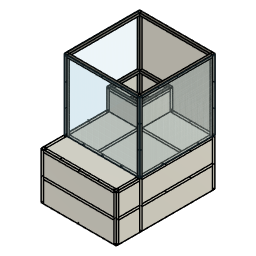
main v17 (Autodesk Fusion 360 design; units mm, degrees)
Autodesk Fusion 360 part; units mm, degrees
note: some values were not read from the file. Chosen so that the rebuilt part matches the saved one: which bodies a step acts on; which face or edge a step refers to.
(part 1 of 2)
sketch "Sketch1" plane through (0, 0, 0) normal (0, 0, 1) x (1, 0, 0) in component "Frame"
  line L0 (0, 0) -> (640, 0)
  line L1 (640, 0) -> (640, 640)
  line L2 (640, 640) -> (0, 640)
  line L3 (0, 640) -> (0, 0)
  line L4 (20, 640) -> (20, 0)
  line L5 (0, 20) -> (640, 20)
  line L6 (620, 640) -> (620, 0)
  line L7 (640, 620) -> (0, 620)
  line L8 (0, 0) -> (0, -200)
  line L9 (0, -200) -> (640, -200)
  line L10 (640, -200) -> (640, 0)
  line L11 (20, 0) -> (20, -200)
  line L12 (620, 0) -> (620, -200)
  line L13 (0, -180) -> (640, -180)
  line L14 (270, 620) -> (270, 20) construction
  line L15 (20, 370) -> (620, 370) construction
  line L16 (280, 620) -> (280, 20)
  line L17 (260, 620) -> (260, 20)
  line L18 (20, 380) -> (620, 380)
  line L19 (20, 360) -> (620, 360)
  line L20 (20, 380) -> (0, 380)
  line L21 (20, 360) -> (0, 360)
  line L22 (260, 620) -> (260, 640)
  line L23 (280, 620) -> (280, 640)
  dimension "d44" = 640
  dimension "d45" = 20
  dimension "d46" = 20
  dimension "d47" = 20
  dimension "d48" = 20
  dimension "d54" = 200
  dimension "d55" = 20
  dimension "d64" = 10
  dimension "d65" = 10
  dimension "d66" = 10
  dimension "d67" = 20
  dimension "d95" = 250
  dimension "d96" = 250
  constraint horizontal L0
  constraint vertical L1
  constraint horizontal L2
  constraint vertical L3
  constraint coincident L0.start L3.end
  constraint equal L0 L3
  constraint coincident L2 L4.start
  constraint coincident L0 L4.end
  constraint perpendicular L0 L4
  constraint coincident L3 L5.start
  constraint coincident L1 L5.end
  constraint perpendicular L1 L5
  constraint coincident L2 L6.start
  constraint coincident L0 L6.end
  constraint perpendicular L0 L6
  constraint coincident L1 L7.start
  constraint coincident L3 L7.end
  constraint perpendicular L3 L7
  constraint vertical L8
  constraint perpendicular L8 L9
  constraint vertical L10
  constraint coincident L9 L11.end
  constraint perpendicular L9 L11
  constraint coincident L9 L12.end
  constraint perpendicular L9 L12
  constraint coincident L8 L13.start
  constraint coincident L10 L13.end
  constraint perpendicular L10 L13
  constraint coincident L7 L16.start
  constraint coincident L5 L16.end
  constraint perpendicular L5 L16
  constraint coincident L7 L17.start
  constraint coincident L5 L17.end
  constraint perpendicular L5 L17
  constraint coincident L4 L18.start
  constraint coincident L6 L18.end
  constraint perpendicular L6 L18
  constraint coincident L4 L19.start
  constraint coincident L6 L19.end
  constraint perpendicular L6 L19
  constraint coincident L4 L15.start
  constraint coincident L6 L15.end
  constraint coincident L5 L14.end
  constraint coincident L7 L14.start
  constraint coincident L3 L20.end
  constraint perpendicular L3 L20
  constraint coincident L3 L21.end
  constraint perpendicular L3 L21
  constraint coincident L2 L22.end
  constraint perpendicular L2 L22
  constraint coincident L2 L23.end
  constraint perpendicular L2 L23
  measures "d44" distance of L0.start L2.end
  measures "d45" distance of L2 L7
  measures "d46" distance of L0 L5
  measures "d47" distance of L3 L4
  measures "d48" distance of L1 L6
  measures "d54" distance of L0.start L8.end
  measures "d55" distance of L9 L13
  measures "d64" distance of L15 L19
  measures "d65" distance of L15 L18
  measures "d66" distance of L14 L16
  measures "d67" distance of L16 L17
  measures "d95" distance of L4 L14
  measures "d96" distance of L7 L15
extrude "Extrude1" add sketch "Sketch1" along normal blind 1000 contours L0 L3 L4 L5 | L0 L1 L5 L6 | L2 L3 L4 L7 | L1 L2 L6 L7 makes body 1 at (0, 633.3333, 333.3333) makes body 2 at (633.3333, 620, 333.3333) makes body 3 at (0, 13.3333, 333.3333) makes body 4 at (620, 13.3333, 333.3333) in component "Frame"
extrude "Extrude6" add sketch "Sketch1" against normal blind 20 from surface at 1000 separate body contours L3 L4 L5 L21 | L3 L4 L20 L21 | L3 L4 L7 L20 makes body 5 in component "Frame"
extrude "Extrude7" add sketch "Sketch1" against normal blind 20 from surface at 1000 separate body contours L2 L4 L7 L22 | L2 L6 L7 L23 | L2 L7 L22 L23 makes body 6 in component "Frame"
extrude "Extrude8" add sketch "Sketch1" against normal blind 20 from surface at 1000 separate body contours L1 L5 L6 L7 makes body 7 in component "Frame"
extrude "Extrude9" add sketch "Sketch1" against normal blind 20 from surface at 1000 separate body contours L0 L4 L5 L6 makes body 8 in component "Frame"
extrude "Extrude3" add sketch "Sketch1" along normal blind 400 separate body contours L8 L9 L11 L13 | L9 L10 L12 L13 makes body 9 at (6.6667, -180, 133.3333) makes body 10 at (640, -193.3333, 133.3333) in component "Frame"
extrude "Extrude5" add sketch "Sketch1" against normal blind 20 from surface at 200 separate body contours L0 L8 L11 L13 | L0 L10 L12 L13 | L9 L11 L12 L13 | L1 L5 L6 L7 makes body 11 at (420, -193.3333, 200) makes body 11 at (20, -60, 193.3333) makes body 11 at (620, -60, 193.3333) makes body 12 at (620, 420, 193.3333) in component "Frame"
extrude "Extrude10" add sketch "Sketch1" against normal blind 20 from surface at 400 separate body contours L0 L8 L11 L13 | L3 L4 L5 L21 | L0 L10 L12 L13 | L3 L4 L20 L21 | L1 L5 L6 L7 | L3 L4 L7 L20 makes body 13 at (640, -120, 393.3333) makes body 14 at (620, 420, 393.3333) makes body 15 at (20, -60, 393.3333) makes body 16 at (20, 420, 393.3333) in component "Frame"
extrude "Extrude11" add sketch "Sketch1" against normal blind 20 from surface at 400 separate body contours L0 L4 L5 L6 | L9 L11 L12 L13 | L2 L4 L7 L22 | L2 L6 L7 L23 | L2 L7 L22 L23 makes body 17 at (420, -193.3333, 400) makes body 18 at (220, 20, 393.3333) makes body 19 at (220, 633.3333, 400) in component "Frame"
extrude "Extrude12" add sketch "Sketch1" against normal blind 20 from surface at 400 separate body contours L5 L16 L17 L19 | L16 L17 L18 L19 | L7 L16 L17 L18 makes body 20 in component "Frame"
extrude "Extrude13" add sketch "Sketch1" against normal blind 20 from surface at 400 separate body contours L4 L17 L18 L19 | L6 L16 L18 L19 makes body 21 at (100, 380, 393.3333) makes body 22 at (393.3333, 360, 393.3333) in component "Frame"
extrude "Extrude16" add sketch "Sketch1" along normal blind 175 from surface at 401 separate body contours L16 L17 L18 L19 makes body 23 in component "Frame"
extrude "Extrude17" add sketch "Sketch1" against normal blind 175 from surface at 576 separate body contours L3 L4 L20 L21 | L2 L7 L22 L23 makes body 24 at (0, 373.3333, 517.6667) makes body 25 at (260, 626.6667, 517.6667) in component "Frame"
extrude "Extrude18" add sketch "Sketch1" against normal blind 20 from surface at 576 separate body contours L4 L17 L18 L19 | L2 L4 L7 L22 makes body 26 at (100, 380, 569.3333) makes body 27 at (100, 633.3333, 576) in component "Frame"
extrude "Extrude19" add sketch "Sketch1" against normal blind 20 from surface at 576 separate body contours L3 L4 L7 L20 | L7 L16 L17 L18 makes body 28 at (260, 540, 569.3333) makes body 29 at (0, 540, 569.3333) in component "Frame"
extrude "Extrude20" add sketch "Sketch1" along normal blind 1 from surface at 400 separate body contours L0 L8 L11 L13 | L0 L4 L5 L6 | L0 L11 L12 L13 | L3 L4 L5 L21 | L8 L9 L11 L13 | L0 L10 L12 L13 | L4 L5 L17 L19 | L9 L11 L12 L13 | L3 L4 L20 L21 | L1 L5 L6 L7 | L5 L6 L16 L19 | L9 L10 L12 L13 | L4 L17 L18 L19 | L5 L16 L17 L19 | L6 L16 L18 L19 | L16 L17 L18 L19 | L6 L7 L16 L18 | L7 L16 L17 L18 | L2 L6 L7 L23 | L2 L7 L22 L23 makes body 30 in component "Frame"
sketch "Sketch3" plane through (0, 360, 0) normal (0, -1, 0) x (1, 0, 0) in component "Frame"
  line L0 (20, 576) -> (0, 576)
  line L1 (0, 576) -> (0, 401)
  line L2 (0, 401) -> (20, 401)
  line L3 (20, 401) -> (20, 576)
  line L4 (0, 576) -> (280, 576)
  line L5 (280, 576) -> (280, 401)
  line L6 (280, 401) -> (0, 401)
  line L7 (0, 401) -> (0, 576)
  dimension "d117" = 280
  dimension "d118" = 175
  constraint horizontal L4
  constraint vertical L5
  constraint horizontal L6
  constraint vertical L7
  constraint coincident L0.end L1.start
  measures "d117" distance of L0.end L4.end
  measures "d118" distance of L0.end L1.end
extrude "Extrude21" add sketch "Sketch3" along normal blind 1 separate body makes body 31 in component "Frame"
sketch "Sketch4" plane through (280, 0, 0) normal (1, 0, 0) x (0, 1, 0) in component "Frame"
  line L0 (360, 401) -> (380, 401)
  line L1 (380, 401) -> (380, 576)
  line L2 (380, 576) -> (360, 576)
  line L3 (360, 576) -> (360, 401)
  line L4 (360, 576) -> (640, 576)
  line L5 (640, 576) -> (640, 401)
  line L6 (640, 401) -> (360, 401)
  line L7 (360, 401) -> (360, 576)
  dimension "d121" = 280
  dimension "d122" = 175
  constraint horizontal L4
  constraint vertical L5
  constraint horizontal L6
  constraint vertical L7
  constraint coincident L2.end L3.start
  measures "d121" distance of L2.end L4.end
  measures "d122" distance of L2.end L0.start
extrude "Extrude22" add sketch "Sketch4" along normal blind 1 separate body makes body 32 in component "Frame"
sketch "Sketch5" plane through (0, 640, 0) normal (0, 1, 0) x (-1, 0, 0) in component "Frame"
  line L0 (-640, 0) -> (-620, 0)
  line L1 (-620, 0) -> (-620, 1000)
  line L2 (-620, 1000) -> (-640, 1000)
  line L3 (-640, 1000) -> (-640, 0)
  line L4 (-640, 1000) -> (0, 1000)
  line L5 (0, 1000) -> (0, 0)
  line L6 (0, 0) -> (-640, 0)
  line L7 (-640, 0) -> (-640, 1000)
  constraint horizontal L4
  constraint vertical L5
  constraint horizontal L6
  constraint vertical L7
  constraint coincident L5.end L6.start
  constraint coincident L2.end L3.start
extrude "Extrude23" add sketch "Sketch5" along normal blind 1 separate body makes body 33 in component "Frame"
sketch "Sketch6" plane through (0, -200, 0) normal (0, -1, 0) x (1, 0, 0) in component "Frame"
  line L0 (0, 0) -> (20, 0)
  line L1 (20, 0) -> (20, 400)
  line L2 (20, 400) -> (0, 400)
  line L3 (0, 400) -> (0, 0)
  line L4 (0, 400) -> (640, 400)
  line L5 (640, 400) -> (640, 0)
  line L6 (640, 0) -> (0, 0)
  line L7 (0, 0) -> (0, 400)
  dimension "d127" = 640
  dimension "d128" = 400
  constraint horizontal L4
  constraint vertical L5
  constraint horizontal L6
  constraint vertical L7
  constraint coincident L2.end L3.start
  measures "d127" distance of L2.end L4.end
  measures "d128" distance of L2.end L0.start
extrude "Extrude24" add sketch "Sketch6" along normal blind 1 separate body makes body 34 in component "Frame"
sketch "Sketch7" plane through (640, 0, 0) normal (1, 0, 0) x (0, 1, 0) in component "Frame"
  line L0 (-200, 0) -> (-180, 0)
  line L1 (-180, 0) -> (-180, 400)
  line L2 (-180, 400) -> (-200, 400)
  line L3 (-200, 400) -> (-200, 0)
  line L4 (-200, 400) -> (640, 400)
  line L5 (640, 400) -> (640, 0)
  line L6 (640, 0) -> (-200, 0)
  line L7 (-200, 0) -> (-200, 400)
  dimension "d131" = 840
  dimension "d132" = 400
  constraint horizontal L4
  constraint vertical L5
  constraint horizontal L6
  constraint vertical L7
  constraint coincident L2.end L3.start
  measures "d131" distance of L2.end L4.end
  measures "d132" distance of L2.end L0.start
extrude "Extrude25" add sketch "Sketch7" along normal blind 1 separate body makes body 35 in component "Frame"
extrude "Extrude26" add sketch "Sketch1" along normal blind 380 separate body contours L3 L4 L20 L21 makes body 36 in component "Frame"
extrude "Extrude27" add sketch "Sketch1" along normal blind 20 from surface at 180 separate body contours L3 L4 L5 L21 | L3 L4 L7 L20 makes body 37 at (0, 246.6667, 186.6667) makes body 38 at (0, 540, 186.6667) in component "Frame"
sketch "Sketch8" plane through (0, 0, 0) normal (-1, 0, 0) x (0, -1, 0) in component "Frame"
  line L0 (-620, 180) -> (-380, 180)
  line L1 (-380, 180) -> (-380, 200)
  line L2 (-380, 200) -> (-620, 200)
  line L3 (-620, 200) -> (-620, 180)
  line L4 (-380, 180) -> (-640, 180)
  line L5 (-640, 180) -> (-640, 0)
  line L6 (-640, 0) -> (-380, 0)
  line L7 (-380, 0) -> (-380, 180)
  line L8 (-640, 0) -> (200, 0)
  line L9 (200, 0) -> (200, 400)
  line L10 (200, 400) -> (-640, 400)
  line L11 (-640, 400) -> (-640, 0)
  line L12 (-640, 400) -> (-360, 400)
  line L13 (-360, 400) -> (-360, 576)
  line L14 (-360, 576) -> (-640, 576)
  line L15 (-640, 576) -> (-640, 400)
  point P0 (-380, 0)
  point P1 (-640, 0)
  point P2 (200, 400)
  point P3 (-360, 576)
  constraint horizontal L4
  constraint vertical L5
  constraint horizontal L6
  constraint vertical L7
  constraint coincident L0.end L1.start
  constraint coincident P0 L6.end
  constraint coincident P1 L5.end
  constraint horizontal L8
  constraint vertical L9
  constraint horizontal L10
  constraint vertical L11
  constraint coincident P2 L9.end
  constraint horizontal L12
  constraint vertical L13
  constraint horizontal L14
  constraint vertical L15
  constraint coincident P3 L13.end
extrude "Extrude28" add sketch "Sketch8" along normal blind 1 separate body contours L0 L1 L2 L3 L4 | L1 L2 L3 L4 L7 L8 L9 L10 L11 L12 | L10 L12 L13 L14 L15 makes body 39 in component "Frame"
extrude "Extrude29" add sketch "Sketch8" along normal blind 1 separate body contours L0 L4 L5 L6 L7 L8 L11 makes body 40 in component "Frame"
sketch "Sketch9" plane through (640, 0, 0) normal (1, 0, 0) x (0, 1, 0) in component "Frame"
  line L0 (620, 0) -> (640, 0)
  line L1 (640, 0) -> (640, 1000)
  line L2 (640, 1000) -> (620, 1000)
  line L3 (620, 1000) -> (620, 0)
  line L4 (640, 1000) -> (0, 1000)
  line L5 (0, 1000) -> (0, 400)
  line L6 (0, 400) -> (640, 400)
  line L7 (640, 400) -> (640, 1000)
  line L8 (0, 0) -> (0, 1000)
  line L9 (-200, 400) -> (640, 400)
  constraint horizontal L4
  constraint vertical L5
  constraint horizontal L6
  constraint vertical L7
  constraint coincident L1.end L2.start
  constraint coincident L5.end L8
  constraint coincident L5.end L9
extrude "Extrude30" add sketch "Sketch9" along normal blind 3 separate body contours L3 L4 L5 L6 L8 L9 | L1 L2 L3 L4 L6 L7 L9 makes body 41 in component "Frame"
extrude "Extrude32" add 1 faces at (643, 206.6667, 600) along direction (-1, 0, 0) blind 3 from surface at 643 separate body on bodies 41 makes body 42 in component "Frame"
sketch "Sketch10" plane through (0, 0, 0) normal (0, -1, 0) x (1, 0, 0) in component "Frame"
  line L0 (620, 0) -> (640, 0)
  line L1 (640, 0) -> (640, 1000)
  line L2 (640, 1000) -> (620, 1000)
  line L3 (620, 1000) -> (620, 0)
  line L4 (640, 1000) -> (0, 1000)
  line L5 (0, 1000) -> (0, 401)
  line L6 (0, 401) -> (640, 401)
  line L7 (640, 401) -> (640, 1000)
  point P0 (0, 1000)
  point P1 (0, 401)
  constraint horizontal L4
  constraint vertical L5
  constraint horizontal L6
  constraint vertical L7
  constraint coincident L1.end L2.start
  constraint coincident L5 P0
  constraint coincident P1 L5.end
extrude "Extrude31" add sketch "Sketch10" along normal blind 3 separate body contours L3 L4 L5 L6 | L1 L2 L3 L4 L6 L7 makes body 43 in component "Frame"
split "Split1" by plane through (620, -180, 200) normal (0, -1, 0) bodies 11 makes body 44 at (620, -60, 193.3333) makes body 45 at (420, -193.3333, 200) in component "Frame"
sketch "Sketch16" plane through (0, 641, 0) normal (0, 1, 0) x (-1, 0, 0) in component "Frame"
  line L0 (-640, 0) -> (0, 0)
  line L1 (0, 0) -> (0, 1000)
  line L2 (0, 1000) -> (-640, 1000)
  line L3 (-640, 1000) -> (-640, 0)
  line L4 (-630, 10) -> (-10, 10) construction
  line L5 (-10, 10) -> (-10, 990) construction
  line L6 (-10, 990) -> (-630, 990) construction
  line L7 (-630, 990) -> (-630, 10) construction
  circle A0 centre (-630, 990) radius 2.1
  circle A1 centre (-10, 990) radius 2.1
  circle A2 centre (-10, 10) radius 2.1
  circle A3 centre (-630, 10) radius 2.1
  circle A4 centre (-320, 990) radius 2.1
  circle A5 centre (-630, 390) radius 2.1
  circle A6 centre (-320, 390) radius 2.1
  circle A7 centre (-10, 390) radius 2.1
  circle A8 centre (-10, 690) radius 2.1
  circle A9 centre (-630, 690) radius 2.1
  dimension "d231" = -10
  dimension "d232" = 4.2
  dimension "d235" = -600
  dimension "d236" = 0
  dimension "d239" = 300
  dimension "d240" = 0
  constraint coincident L6.end L7.start
  constraint coincident L5.end L6.start
  constraint coincident L4.end L5.start
  constraint coincident L4.start L7.end
  constraint equal A2 A3
  constraint equal A1 A2
  constraint equal A0 A1
  constraint midpoint L6 A4.centre
  constraint equal A1 A4
  measures "d232" diameter of A0
extrude "Extrude38" cut sketch "Sketch16" against normal up to surface (1 mm away) contours A0 | A1 | A2 | A3 | A4 | A5 | A6 | A7 | A8 | A9 bodies 33 in component "Frame"
sketch "Sketch12" plane through (641, 0, 0) normal (1, 0, 0) x (0, 1, 0) in component "Frame"
  line L0 (-200, 0) -> (640, 0)
  line L1 (640, 0) -> (640, 400)
  line L2 (640, 400) -> (-200, 400)
  line L3 (-200, 400) -> (-200, 0)
  line L4 (-190, 390) -> (630, 390) construction
  line L5 (630, 390) -> (630, 10) construction
  line L6 (630, 10) -> (-190, 10) construction
  line L7 (-190, 10) -> (-190, 390) construction
  circle A0 centre (-190, 390) radius 2.1
  circle A1 centre (10, 390) radius 2.1
  circle A2 centre (630, 390) radius 2.1
  circle A3 centre (220, 390) radius 2.1
  circle A4 centre (430, 390) radius 2.1
  circle A5 centre (-190, 190) radius 2.1
  circle A6 centre (10, 190) radius 2.1
  circle A7 centre (630, 190) radius 2.1
  circle A8 centre (10, 10) radius 2.1
  circle A9 centre (630, 10) radius 2.1
  circle A10 centre (-190, 10) radius 2.1
  circle A11 centre (430, 190) radius 2.1
  circle A12 centre (220, 190) radius 2.1
  dimension "d170" = 10
  dimension "d171" = 10
  dimension "d172" = 10
  dimension "d173" = 10
  dimension "d174" = 4.2
  dimension "d175" = 200
  dimension "d176" = 200
  dimension "d180" = -200
  dimension "d181" = 0
  dimension "d184" = -180
  dimension "d185" = 0
  dimension "d190" = 0
  dimension "d191" = -200
  constraint horizontal L4
  constraint vertical L5
  constraint horizontal L6
  constraint vertical L7
  constraint coincident L4.start L7.end
  constraint coincident L4 A1.centre
  constraint equal A0 A1
  constraint coincident L4.end L5.start
  constraint equal A1 A2
  constraint coincident L4 A3.centre
  constraint coincident L4 A4.centre
  constraint midpoint L4 A3.centre
  constraint equal A3 A4
  constraint equal A2 A4
  measures "d170" distance of L2 L4
  measures "d171" distance of L3 L7
  measures "d172" distance of L1 L5
  measures "d173" distance of L0 L6
  measures "d174" diameter of A0
  measures "d175" distance of L4.start A1.centre
  measures "d176" distance of L4.end A4.centre
extrude "Extrude34" cut sketch "Sketch12" against normal blind 1 contours A0 | A1 | A2 | A3 | A4 | A5 | A6 | A7 | A8 | A9 | A10 | A11 | A12 bodies 35 in component "Frame"
sketch "Sketch13" plane through (0, 359, 0) normal (0, -1, 0) x (1, 0, 0) in component "Frame"
  line L0 (0, 401) -> (280, 401)
  line L1 (280, 401) -> (280, 576)
  line L2 (280, 576) -> (0, 576)
  line L3 (0, 576) -> (0, 401)
  line L4 (10, 411) -> (270, 411) construction
  line L5 (270, 411) -> (270, 566) construction
  line L6 (270, 566) -> (10, 566) construction
  line L7 (10, 566) -> (10, 411) construction
  circle A0 centre (10, 566) radius 2.1
  circle A1 centre (270, 566) radius 2.1
  circle A2 centre (270, 411) radius 2.1
  circle A3 centre (10, 411) radius 2.1
  dimension "d192" = -10
  dimension "d193" = 4.2
  constraint coincident L6.end L7.start
  constraint coincident L5.end L6.start
  constraint coincident L4.end L5.start
  constraint coincident L4.start L7.end
  constraint equal A0 A1
  constraint equal A1 A2
  constraint equal A2 A3
  measures "d193" diameter of A0
extrude "Extrude35" cut sketch "Sketch13" against normal up to surface (1 mm away) contours A0 | A1 | A2 | A3 bodies 31 in component "Frame"
sketch "Sketch14" plane through (281, 0, 0) normal (1, 0, 0) x (0, 1, 0) in component "Frame"
  line L0 (360, 401) -> (640, 401)
  line L1 (640, 401) -> (640, 576)
  line L2 (640, 576) -> (360, 576)
  line L3 (360, 576) -> (360, 401)
  line L4 (370, 411) -> (630, 411) construction
  line L5 (630, 411) -> (630, 566) construction
  line L6 (630, 566) -> (370, 566) construction
  line L7 (370, 566) -> (370, 411) construction
  circle A0 centre (370, 566) radius 2.1
  circle A1 centre (630, 566) radius 2.1
  circle A2 centre (630, 411) radius 2.1
  circle A3 centre (370, 411) radius 2.1
  dimension "d196" = -10
  dimension "d197" = 4.2
  constraint coincident L6.end L7.start
  constraint coincident L5.end L6.start
  constraint coincident L4.end L5.start
  constraint coincident L4.start L7.end
  constraint equal A2 A3
  constraint equal A1 A2
  constraint equal A0 A1
  measures "d197" diameter of A0
extrude "Extrude36" cut sketch "Sketch14" against normal up to surface (1 mm away) contours A0 | A1 | A2 | A3 bodies 32 in component "Frame"
sketch "Sketch15" plane through (0, 0, 401) normal (0, 0, 1) x (-1, 0, 0) in component "Frame"
  line L0 (-260, -380) -> (0, -380)
  line L1 (0, -380) -> (0, -20)
  line L2 (0, -20) -> (-20, -20)
  line L3 (-20, -20) -> (-20, 0)
  line L4 (-20, 0) -> (0, 0)
  line L5 (0, 0) -> (0, 200)
  line L6 (0, 200) -> (-640, 200)
  line L7 (-640, 200) -> (-640, 0)
  line L8 (-640, 0) -> (-620, 0)
  line L9 (-620, 0) -> (-620, -20)
  line L10 (-620, -20) -> (-640, -20)
  line L11 (-640, -20) -> (-640, -620)
  line L12 (-640, -620) -> (-620, -620)
  line L13 (-620, -620) -> (-620, -640)
  line L14 (-620, -640) -> (-260, -640)
  line L15 (-260, -640) -> (-260, -380)
  line L16 (0, -380) -> (-20, -380) construction
  line L17 (-20, -380) -> (-20, -360) construction
  line L18 (-20, -360) -> (0, -360) construction
  line L19 (0, -360) -> (0, -380) construction
  line L20 (-260, -380) -> (-280, -380) construction
  line L21 (-280, -380) -> (-280, -360) construction
  line L22 (-280, -360) -> (-260, -360) construction
  line L23 (-260, -360) -> (-260, -380) construction
  line L24 (-260, -640) -> (-280, -640) construction
  line L25 (-280, -640) -> (-280, -620) construction
  line L26 (-280, -620) -> (-260, -620) construction
  line L27 (-260, -620) -> (-260, -640) construction
  line L28 (-10, -30) -> (-30, -30) construction
  line L29 (-30, -30) -> (-30, 10) construction
  line L30 (-30, 10) -> (-10, 10) construction
  line L31 (-10, 10) -> (-10, 190) construction
  line L32 (-10, 190) -> (-630, 190) construction
  line L33 (-630, 190) -> (-630, 10) construction
  line L34 (-630, 10) -> (-610, 10) construction
  line L35 (-610, 10) -> (-610, -30) construction
  line L36 (-610, -30) -> (-630, -30) construction
  line L37 (-630, -30) -> (-630, -610) construction
  line L38 (-630, -610) -> (-610, -610) construction
  line L39 (-610, -610) -> (-610, -630) construction
  line L40 (-610, -630) -> (-270, -630) construction
  line L41 (-270, -630) -> (-270, -370) construction
  line L42 (-270, -370) -> (-10, -370) construction
  line L43 (-10, -370) -> (-10, -30) construction
  circle A0 centre (-10, -349) radius 2.1
  circle A1 centre (-31, -370) radius 2.1
  circle A2 centre (-249, -370) radius 2.1
  circle A3 centre (-270, -391) radius 2.1
  circle A4 centre (-270, -609) radius 2.1
  circle A5 centre (-291, -630) radius 2.1
  circle A6 centre (-609, -630) radius 2.1
  circle A7 centre (-630, -609) radius 2.1
  circle A8 centre (-630, -31) radius 2.1
  circle A9 centre (-630, 11) radius 2.1
  circle A10 centre (-10, 11) radius 2.1
  circle A11 centre (-10, -31) radius 2.1
  circle A12 centre (-440, -630) radius 2.1
  circle A13 centre (-270, -500) radius 2.1
  circle A14 centre (-140, -370) radius 2.1
  circle A15 centre (-10, -200) radius 2.1
  circle A16 centre (-630, -200) radius 2.1
  circle A17 centre (-630, -500) radius 2.1
  line L44 (0, 200) -> (-20, 200) construction
  line L45 (-20, 200) -> (-20, 180) construction
  line L46 (-20, 180) -> (0, 180) construction
  line L47 (0, 180) -> (0, 200) construction
  line L48 (-640, 200) -> (-620, 200) construction
  line L49 (-620, 200) -> (-620, 180) construction
  line L50 (-620, 180) -> (-640, 180) construction
  line L51 (-640, 180) -> (-640, 200) construction
  circle A18 centre (-630, 170) radius 2.1
  circle A19 centre (-610, 190) radius 2.1
  circle A20 centre (-30, 190) radius 2.1
  circle A21 centre (-10, 170) radius 2.1
  circle A22 centre (-320, 190) radius 2.1
  circle A23 centre (-160, 190) radius 2.1
  circle A24 centre (-480, 190) radius 2.1
  line L52 (-20, -10) -> (-620, -10) construction
  circle A25 centre (-31, -10) radius 2.1
  circle A26 centre (-609, -10) radius 2.1
  circle A27 centre (-160, -10) radius 2.1
  circle A28 centre (-320, -10) radius 2.1
  circle A29 centre (-480, -10) radius 2.1
  line L53 (0, -21) -> (-21, -21)
  line L54 (-21, -21) -> (-21, 1)
  line L55 (-21, 1) -> (0, 1)
  line L56 (0, 1) -> (0, -21)
  line L57 (-640, -21) -> (-619, -21)
  line L58 (-619, -21) -> (-619, 1)
  line L59 (-619, 1) -> (-640, 1)
  line L60 (-619, -640) -> (-619, -619)
  line L61 (-619, -619) -> (-640, -619)
  dimension "d200" = 20
  dimension "d201" = -10
  dimension "d202" = 4.2
  dimension "d203" = 11
  dimension "d204" = 11
  dimension "d205" = 11
  dimension "d206" = 11
  dimension "d207" = 11
  dimension "d208" = 11
  dimension "d209" = 11
  dimension "d210" = 11
  dimension "d211" = 11
  dimension "d212" = 11
  dimension "d213" = 11
  dimension "d214" = 11
  dimension "d215" = 20
  dimension "d216" = 20
  dimension "d217" = 20
  dimension "d218" = 20
  dimension "d219" = 20
  dimension "d220" = 20
  dimension "d221" = 130
  dimension "d222" = 130
  dimension "d223" = 11
  dimension "d224" = 11
  dimension "d227" = 0
  dimension "d228" = -200
  dimension "d272" = 1
  dimension "d273" = 1
  dimension "d274" = 1
  dimension "d275" = 1
  dimension "d276" = 1
  dimension "d277" = 1
  dimension "d278" = 1
  dimension "d279" = 1
  constraint horizontal L16
  constraint vertical L17
  constraint horizontal L18
  constraint vertical L19
  constraint coincident L0.end L1.start
  constraint equal L17 L18
  constraint horizontal L20
  constraint vertical L21
  constraint horizontal L22
  constraint vertical L23
  constraint coincident L0.start L15.end
  constraint equal L20 L21
  constraint equal L17 L21
  constraint horizontal L24
  constraint vertical L25
  constraint horizontal L26
  constraint vertical L27
  constraint coincident L14.end L15.start
  constraint equal L25 L26
  constraint equal L20 L26
  constraint coincident L43 A0.centre
  constraint coincident L42 A1.centre
  constraint coincident L42 A2.centre
  constraint coincident L41 A3.centre
  constraint coincident L41 A4.centre
  constraint coincident L40 A5.centre
  constraint coincident L40 A6.centre
  constraint coincident L37 A7.centre
  constraint coincident L37 A8.centre
  constraint coincident L33 A9.centre
  constraint coincident L31 A10.centre
  constraint coincident L43 A11.centre
  constraint equal A0 A1
  constraint equal A1 A10
  constraint equal A10 A11
  constraint equal A9 A11
  constraint equal A8 A9
  constraint equal A2 A8
  constraint equal A2 A3
  constraint equal A3 A4
  constraint equal A4 A5
  constraint equal A5 A7
  constraint equal A6 A7
  constraint midpoint L40 A12.centre
  constraint midpoint L41 A13.centre
  constraint midpoint L42 A14.centre
  constraint midpoint L43 A15.centre
  constraint coincident L37 A16.centre
  constraint horizontal A15.centre A16.centre
  constraint coincident L37 A17.centre
  constraint horizontal A13.centre A17.centre
  constraint equal A16 A17
  constraint equal A12 A17
  constraint equal A12 A13
  constraint equal A13 A14
  constraint equal A14 A15
  constraint equal A0 A15
  constraint horizontal L44
  constraint vertical L45
  constraint horizontal L46
  constraint vertical L47
  constraint coincident L5.end L6.start
  constraint horizontal L48
  constraint vertical L49
  constraint horizontal L50
  constraint vertical L51
  constraint coincident L6.end L7.start
  constraint equal L49 L50
  constraint equal L45 L49
  constraint coincident L33 A18.centre
  constraint coincident L32 A19.centre
  constraint coincident L32 A20.centre
  constraint coincident L31 A21.centre
  constraint midpoint L32 A22.centre
  constraint coincident L32 A23.centre
  constraint coincident L32 A24.centre
  constraint equal A20 A21
  constraint equal A20 A23
  constraint equal A22 A23
  constraint equal A22 A24
  constraint equal A19 A24
  constraint equal A18 A19
  constraint equal A9 A18
  constraint midpoint L3 L52.start
  constraint midpoint L9 L52.end
  constraint coincident L52 A25.centre
  constraint coincident L52 A26.centre
  constraint equal A25 A26
  constraint equal A8 A26
  constraint horizontal L53
  constraint vertical L54
  constraint horizontal L55
  constraint vertical L56
  constraint coincident L1.end L56
  constraint coincident L11 L57.start
  constraint perpendicular L11 L57
  constraint perpendicular L10 L58
  constraint coincident L7 L59.end
  constraint perpendicular L7 L59
  constraint coincident L14 L60.start
  constraint perpendicular L14 L60
  constraint coincident L11 L61.end
  constraint perpendicular L11 L61
  measures "d200" distance of L0.end L16.end
  measures "d202" diameter of A0
  measures "d203" distance of L18 A0.centre
  measures "d204" distance of L17 A1.centre
  measures "d205" distance of L2 A11.centre
  measures "d206" distance of L4 A10.centre
  measures "d207" distance of L8 A9.centre
  measures "d208" distance of L10 A8.centre
  measures "d209" distance of L12 A7.centre
  measures "d210" distance of L13 A6.centre
  measures "d211" distance of L25 A5.centre
  measures "d212" distance of L26 A4.centre
  measures "d213" distance of L20 A3.centre
  measures "d214" distance of L23 A2.centre
  measures "d215" distance of L5.end L44.end
  measures "d216" distance of L5.end L46.end
  measures "d217" distance of L32.end A18.centre
  measures "d218" distance of L31.end A20.centre
  measures "d219" distance of L31.end A21.centre
  measures "d220" distance of L32.end A19.centre
  measures "d221" distance of A19.centre A24.centre
  measures "d222" distance of A20.centre A23.centre
  measures "d223" distance of L52.end A26.centre
  measures "d224" distance of L3 A25.centre
  measures "d272" distance of L2 L53
  measures "d273" distance of L4 L55
  measures "d274" distance of L3 L54
  measures "d275" distance of L8 L59
  measures "d276" distance of L10 L57
  measures "d277" distance of L9 L58
  measures "d278" distance of L12 L61
  measures "d279" distance of L13 L60
extrude "Extrude37" cut sketch "Sketch15" against normal up to surface (1 mm away) contours L1 L2 L3 L4 L5 L53 L54 L55 L56 | L11 L12 L13 L14 L60 L61 | L7 L8 L9 L10 L11 L57 L58 L59 | A0 | A1 | A2 | A3 | A4 | A5 | A6 | A7 | A8 | A9 | A10 | A11 | A12 | A13 | A14 | A15 | A16 | A17 | A18 | A19 | A20 | A21 | A22 | A23 | A24 | A25 | A26 | A27 | A28 | A29 bodies 30 in component "Frame"
sketch "Sketch17" plane through (-1, 0, 0) normal (-1, 0, 0) x (0, -1, 0) in component "Frame"
  line L0 (-380, 0) -> (200, 0)
  line L1 (200, 0) -> (200, 400)
  line L2 (200, 400) -> (-360, 400)
  line L3 (-360, 400) -> (-360, 576)
  line L4 (-360, 576) -> (-640, 576)
  line L5 (-640, 576) -> (-640, 180)
  line L6 (-640, 180) -> (-380, 180)
  line L7 (-380, 180) -> (-380, 0)
  line L8 (190, 10) -> (190, 390) construction
  line L9 (190, 390) -> (-370, 390) construction
  line L10 (-370, 390) -> (-370, 566) construction
  line L11 (-370, 566) -> (-630, 566) construction
  line L12 (-630, 566) -> (-630, 190) construction
  line L13 (-630, 190) -> (-370, 190) construction
  line L14 (-370, 190) -> (-370, 10) construction
  line L15 (-370, 10) -> (190, 10) construction
  circle A0 centre (-630, 566) radius 2.1
  circle A1 centre (-370, 566) radius 2.1
  circle A2 centre (-370, 390) radius 2.1
  circle A3 centre (-630, 190) radius 2.1
  circle A4 centre (-370, 190) radius 2.1
  circle A5 centre (-370, 10) radius 2.1
  circle A6 centre (190, 10) radius 2.1
  circle A7 centre (190, 390) radius 2.1
  circle A8 centre (-630, 390) radius 2.1
  circle A9 centre (-10, 10) radius 2.1
  circle A10 centre (-10, 390) radius 2.1
  circle A11 centre (190, 190) radius 2.1
  circle A12 centre (-10, 190) radius 2.1
  circle A13 centre (-370, 410) radius 2.1
  circle A14 centre (-630, 410) radius 2.1
  dimension "d243" = -10
  dimension "d244" = 4.2
  dimension "d247" = 200
  dimension "d252" = 20
  constraint coincident L11.end L12.start
  constraint coincident L10.end L11.start
  constraint coincident L9.end L10.start
  constraint coincident L12.end L13.start
  constraint coincident L13.end L14.start
  constraint coincident L14.end L15.start
  constraint coincident L8.start L15.end
  constraint coincident L8.end L9.start
  constraint coincident L12 A8.centre
  constraint horizontal L9.end A8.centre
  constraint coincident L9 A10.centre
  constraint vertical A9.centre A10.centre
  constraint equal A6 A9
  constraint equal A5 A9
  constraint equal A4 A5
  constraint equal A4 A10
  constraint equal A2 A10
  constraint equal A2 A3
  constraint equal A3 A8
  constraint equal A1 A8
  constraint equal A0 A1
  constraint equal A0 A7
  constraint coincident L8 A11.centre
  constraint horizontal L13.end A11.centre
  constraint equal A7 A11
  constraint vertical A9.centre A12.centre
  constraint horizontal A11.centre A12.centre
  constraint equal A11 A12
  constraint coincident L10 A13.centre
  constraint coincident L12 A14.centre
  constraint equal A13 A14
  constraint equal A2 A13
  constraint horizontal A13.centre A14.centre
  measures "d244" diameter of A7
  measures "d247" distance of L8.end A10.centre
  measures "d252" distance of L9.end A13.centre
extrude "Extrude39" cut sketch "Sketch17" against normal up to surface (1 mm away) contours A0 | A1 | A3 | A4 | A5 | A6 | A7 | A9 | A10 | A11 | A12 | A13 | A14 bodies 39 in component "Frame"
sketch "Sketch18" plane through (0, -201, 0) normal (0, -1, 0) x (1, 0, 0) in component "Frame"
  line L0 (0, 0) -> (640, 0)
  line L1 (640, 0) -> (640, 400)
  line L2 (640, 400) -> (0, 400)
  line L3 (0, 400) -> (0, 0)
  line L4 (630, 10) -> (630, 390) construction
  line L5 (630, 390) -> (10, 390) construction
  line L6 (10, 390) -> (10, 10) construction
  line L7 (10, 10) -> (630, 10) construction
  circle A0 centre (10, 390) radius 2.1
  circle A1 centre (320, 390) radius 2.1
  circle A2 centre (630, 390) radius 2.1
  circle A3 centre (10, 10) radius 2.1
  circle A4 centre (320, 10) radius 2.1
  circle A5 centre (630, 10) radius 2.1
  circle A6 centre (10, 200) radius 2.1
  circle A7 centre (630, 200) radius 2.1
  line L8 (10, 200) -> (630, 200) construction
  circle A8 centre (320, 200) radius 2.1
  dimension "d248" = -10
  dimension "d249" = 4.2
  constraint coincident L5.end L6.start
  constraint midpoint L5 A1.centre
  constraint coincident L4.end L5.start
  constraint coincident L6.end L7.start
  constraint midpoint L7 A4.centre
  constraint coincident L4.start L7.end
  constraint midpoint L6 A6.centre
  constraint midpoint L4 A7.centre
  constraint equal A5 A7
  constraint equal A4 A5
  constraint equal A3 A4
  constraint equal A3 A6
  constraint equal A0 A6
  constraint equal A0 A1
  constraint equal A1 A2
  constraint coincident A6.centre L8.start
  constraint coincident A7.centre L8.end
  constraint midpoint L8 A8.centre
  constraint equal A1 A8
  measures "d249" diameter of A2
extrude "Extrude40" cut sketch "Sketch18" against normal up to surface (1 mm away) contours A0 | A1 | A2 | A3 | A4 | A5 | A6 | A7 | A8 bodies 34 in component "Frame"
sketch "Sketch19" plane through (0, -3, 0) normal (0, -1, 0) x (1, 0, 0) in component "Frame"
  line L0 (640, 401) -> (640, 1000)
  line L1 (640, 1000) -> (0, 1000)
  line L2 (0, 1000) -> (0, 401)
  line L3 (0, 401) -> (640, 401)
  line L4 (10, 411) -> (630, 411) construction
  line L5 (630, 411) -> (630, 990) construction
  line L6 (630, 990) -> (10, 990) construction
  line L7 (10, 990) -> (10, 411) construction
  circle A0 centre (160, 411) radius 2.1
  circle A1 centre (10, 411) radius 2.1
  circle A2 centre (320, 411) radius 2.1
  circle A3 centre (630, 411) radius 2.1
  circle A4 centre (480, 411) radius 2.1
  circle A5 centre (160, 990) radius 2.1
  circle A6 centre (320, 990) radius 2.1
  circle A7 centre (480, 990) radius 2.1
  circle A8 centre (10, 604) radius 2.1
  circle A9 centre (630, 604) radius 2.1
  circle A10 centre (10, 797) radius 2.1
  circle A11 centre (630, 797) radius 2.1
  circle A12 centre (10, 990) radius 2.1
  circle A13 centre (630, 990) radius 2.1
  dimension "d253" = -10
  dimension "d254" = 150
  dimension "d255" = 150
  dimension "d256" = 4.2
  dimension "d259" = 579
  dimension "d260" = 0
  dimension "d263" = 0
  dimension "d264" = 579
  constraint coincident L4 A0.centre
  constraint coincident L4.start L7.end
  constraint midpoint L4 A2.centre
  constraint coincident L4.end L5.start
  constraint coincident L4 A4.centre
  constraint equal A1 A3
  constraint equal A0 A1
  constraint equal A0 A2
  constraint equal A2 A4
  measures "d254" distance of L4.start A0.centre
  measures "d255" distance of L4.end A4.centre
  measures "d256" diameter of A3
extrude "Extrude41" cut sketch "Sketch19" against normal up to surface (3 mm away) contours A0 | A1 | A2 | A3 | A4 | A5 | A6 | A7 | A8 | A9 | A10 | A11 | A12 | A13 bodies 43 in component "Frame"
sketch "Sketch28" plane through (643, 0, 0) normal (1, 0, 0) x (0, 1, 0) in component "Frame"
  line L0 (640, 400) -> (640, 1000)
  line L1 (640, 1000) -> (0, 1000)
  line L2 (0, 1000) -> (0, 400)
  line L3 (0, 400) -> (640, 400)
  line L4 (10, 410) -> (630, 410) construction
  line L5 (630, 410) -> (630, 990) construction
  line L6 (630, 990) -> (10, 990) construction
  line L7 (10, 990) -> (10, 410) construction
  circle A0 centre (10, 990) radius 2.1
  circle A1 centre (630, 990) radius 2.1
  circle A2 centre (320, 990) radius 2.1
  circle A3 centre (480, 990) radius 2.1
  circle A4 centre (160, 990) radius 2.1
  circle A5 centre (10, 796.6667) radius 2.1
  circle A6 centre (630, 796.6667) radius 2.1
  circle A7 centre (10, 603.3333) radius 2.1
  circle A8 centre (630, 603.3333) radius 2.1
  circle A9 centre (10, 410) radius 2.1
  circle A10 centre (630, 410) radius 2.1
  circle A11 centre (200, 410) radius 2.1
  circle A12 centre (500, 410) radius 2.1
  dimension "d280" = -10
  dimension "d281" = 150
  dimension "d282" = 150
  dimension "d283" = 4.2
  dimension "d286" = 580
  dimension "d287" = 0
  dimension "d288" = 190
  dimension "d289" = 130
  constraint coincident L6.end L7.start
  constraint coincident L5.end L6.start
  constraint midpoint L6 A2.centre
  constraint coincident L6 A3.centre
  constraint coincident L6 A4.centre
  constraint equal A0 A4
  constraint equal A2 A4
  constraint equal A2 A3
  constraint equal A1 A3
  constraint coincident L4 A11.centre
  constraint equal A9 A11
  constraint coincident L4 A12.centre
  constraint equal A10 A12
  measures "d281" distance of L6.end A4.centre
  measures "d282" distance of L5.end A3.centre
  measures "d283" diameter of A1
  measures "d288" distance of L4.start A11.centre
  measures "d289" distance of L4.end A12.centre
extrude "Extrude42" cut sketch "Sketch28" against normal up to surface (3 mm away) contours A0 | A1 | A2 | A3 | A4 | A5 | A6 | A7 | A8 | A9 | A10 | A11 | A12 bodies 41 in component "Frame"
extrude "Extrude43" cut sketch "Sketch28" along normal up to surface (3 mm away) from surface at -646 contours A0 | A1 | A2 | A3 | A4 | A5 | A6 | A7 | A8 | A9 | A10 | A11 bodies 42 in component "Frame"
extrude "Extrude44" cut sketch "Sketch17" along normal up to surface (3 mm away) from surface at -1 contours A0 | A1 | A13 | A14 bodies 42 in component "Frame"
sketch "Pannel_ground" plane through (0, 0, 401) normal (0, 0, 1) x (-1, 0, 0) in component "Frame"
  circle A0 centre (-440, -630) radius 2.1
  circle A1 centre (-10, -200) radius 2.1
  circle A2 centre (-630, -200) radius 2.1
  circle A3 centre (-320, -10) radius 2.1
  circle A4 centre (-480, -10) radius 2.1
  circle A5 centre (-291, -630) radius 2.1
  circle A6 centre (-270, -391) radius 2.1
  circle A7 centre (-630, 11) radius 2.1
  circle A8 centre (-630, -609) radius 2.1
  circle A9 centre (-249, -370) radius 2.1
  circle A10 centre (-160, 190) radius 2.1
  circle A11 centre (-480, 190) radius 2.1
  circle A12 centre (-630, -500) radius 2.1
  circle A13 centre (-610, 190) radius 2.1
  circle A14 centre (-10, 170) radius 2.1
  circle A15 centre (-270, -500) radius 2.1
  circle A16 centre (-630, 170) radius 2.1
  circle A17 centre (-10, -31) radius 2.1
  circle A18 centre (-609, -10) radius 2.1
  circle A19 centre (-160, -10) radius 2.1
  circle A20 centre (-31, -370) radius 2.1
  circle A21 centre (-630, -31) radius 2.1
  circle A22 centre (-270, -609) radius 2.1
  circle A23 centre (-10, -349) radius 2.1
  circle A24 centre (-609, -630) radius 2.1
  circle A25 centre (-320, 190) radius 2.1
  circle A26 centre (-31, -10) radius 2.1
  circle A27 centre (-140, -370) radius 2.1
  circle A28 centre (-30, 190) radius 2.1
  circle A29 centre (-10, 11) radius 2.1
  line L0 (-260, -380) -> (0, -380)
  line L1 (0, -380) -> (0, -21)
  line L2 (0, 1) -> (0, 200)
  line L3 (0, 200) -> (-640, 200)
  line L4 (-640, 200) -> (-640, 1)
  line L5 (-640, -21) -> (-640, -619)
  line L6 (-619, -640) -> (-260, -640)
  line L7 (-260, -640) -> (-260, -380)
  line L8 (0, -21) -> (-21, -21)
  line L9 (-21, -21) -> (-21, 1)
  line L10 (-21, 1) -> (0, 1)
  line L11 (-640, 1) -> (-619, 1)
  line L12 (-619, 1) -> (-619, -21)
  line L13 (-619, -21) -> (-640, -21)
  line L14 (-640, -619) -> (-619, -619)
  line L15 (-619, -619) -> (-619, -640)
sketch "Pannel_front" plane through (0, -201, 0) normal (0, -1, 0) x (1, 0, 0) in component "Frame"
  circle A0 centre (320, 10) radius 2.1
  circle A1 centre (320, 390) radius 2.1
  circle A2 centre (10, 10) radius 2.1
  circle A3 centre (630, 10) radius 2.1
  circle A4 centre (320, 200) radius 2.1
  circle A5 centre (630, 390) radius 2.1
  circle A6 centre (10, 390) radius 2.1
  circle A7 centre (630, 200) radius 2.1
  circle A8 centre (10, 200) radius 2.1
  line L0 (0, 0) -> (640, 0)
  line L1 (640, 0) -> (640, 400)
  line L2 (640, 400) -> (0, 400)
  line L3 (0, 400) -> (0, 0)
sketch "Pannel_right" plane through (641, 0, 0) normal (1, 0, 0) x (0, 1, 0) in component "Frame"
  circle A0 centre (-190, 10) radius 2.1
  circle A1 centre (10, 190) radius 2.1
  circle A2 centre (430, 390) radius 2.1
  circle A3 centre (10, 390) radius 2.1
  circle A4 centre (-190, 190) radius 2.1
  circle A5 centre (10, 10) radius 2.1
  circle A6 centre (220, 190) radius 2.1
  circle A7 centre (-190, 390) radius 2.1
  circle A8 centre (630, 10) radius 2.1
  circle A9 centre (630, 390) radius 2.1
  circle A10 centre (220, 390) radius 2.1
  circle A11 centre (630, 190) radius 2.1
  circle A12 centre (430, 190) radius 2.1
  line L0 (-200, 0) -> (640, 0)
  line L1 (640, 0) -> (640, 400)
  line L2 (640, 400) -> (-200, 400)
  line L3 (-200, 400) -> (-200, 0)
sketch "Pannel_left" plane through (-1, 0, 0) normal (-1, 0, 0) x (0, -1, 0) in component "Frame"
  circle A0 centre (-10, 10) radius 2.1
  circle A1 centre (-630, 190) radius 2.1
  circle A2 centre (190, 10) radius 2.1
  circle A3 centre (-370, 10) radius 2.1
  circle A4 centre (-630, 566) radius 2.1
  circle A5 centre (-10, 190) radius 2.1
  circle A6 centre (-630, 410) radius 2.1
  circle A7 centre (-10, 390) radius 2.1
  circle A8 centre (190, 390) radius 2.1
  circle A9 centre (-370, 190) radius 2.1
  circle A10 centre (-370, 566) radius 2.1
  circle A11 centre (190, 190) radius 2.1
  circle A12 centre (-370, 410) radius 2.1
  line L0 (-380, 0) -> (200, 0)
  line L1 (200, 0) -> (200, 400)
  line L2 (200, 400) -> (-360, 400)
  line L3 (-360, 400) -> (-360, 576)
  line L4 (-360, 576) -> (-640, 576)
  line L5 (-640, 576) -> (-640, 180)
  line L6 (-640, 180) -> (-380, 180)
  line L7 (-380, 180) -> (-380, 0)
sketch "Pannel_door" plane through (-1, 0, 0) normal (-1, 0, 0) x (0, -1, 0) in component "Frame"
  line L0 (-380, 180) -> (-640, 180)
  line L1 (-640, 180) -> (-640, 0)
  line L2 (-640, 0) -> (-380, 0)
  line L3 (-380, 0) -> (-380, 180)
sketch "Pannel_out1" plane through (0, 359, 0) normal (0, -1, 0) x (1, 0, 0) in component "Frame"
  circle A0 centre (10, 566) radius 2.1
  circle A1 centre (270, 566) radius 2.1
  circle A2 centre (10, 411) radius 2.1
  circle A3 centre (270, 411) radius 2.1
  line L0 (0, 401) -> (280, 401)
  line L1 (280, 401) -> (280, 576)
  line L2 (280, 576) -> (0, 576)
  line L3 (0, 576) -> (0, 401)
sketch "Pannel_out2" plane through (281, 0, 0) normal (1, 0, 0) x (0, 1, 0) in component "Frame"
  circle A0 centre (370, 566) radius 2.1
  circle A1 centre (630, 566) radius 2.1
  circle A2 centre (370, 411) radius 2.1
  circle A3 centre (630, 411) radius 2.1
  line L0 (360, 401) -> (640, 401)
  line L1 (640, 401) -> (640, 576)
  line L2 (640, 576) -> (360, 576)
  line L3 (360, 576) -> (360, 401)
sketch "Pannel_back" plane through (0, 641, 0) normal (0, 1, 0) x (-1, 0, 0) in component "Frame"
  circle A0 centre (-10, 10) radius 2.1
  circle A1 centre (-10, 690) radius 2.1
  circle A2 centre (-320, 990) radius 2.1
  circle A3 centre (-320, 390) radius 2.1
  circle A4 centre (-10, 990) radius 2.1
  circle A5 centre (-630, 690) radius 2.1
  circle A6 centre (-10, 390) radius 2.1
  circle A7 centre (-630, 10) radius 2.1
  circle A8 centre (-630, 390) radius 2.1
  circle A9 centre (-630, 990) radius 2.1
  line L0 (-640, 0) -> (0, 0)
  line L1 (0, 0) -> (0, 1000)
  line L2 (0, 1000) -> (-640, 1000)
  line L3 (-640, 1000) -> (-640, 0)
sketch "Sketch4 (2)" plane through (0, -3, 0) normal (0, -1, 0) x (1, 0, 0)
  circle A0 centre (10, 990) radius 2.1
  circle A1 centre (10, 797) radius 2.1
  circle A2 centre (480, 411) radius 2.1
  circle A3 centre (320, 990) radius 2.1
  circle A4 centre (630, 990) radius 2.1
  circle A5 centre (320, 411) radius 2.1
  circle A6 centre (160, 990) radius 2.1
  circle A7 centre (480, 990) radius 2.1
  circle A8 centre (10, 604) radius 2.1
  circle A9 centre (630, 797) radius 2.1
  circle A10 centre (630, 604) radius 2.1
  circle A11 centre (630, 411) radius 2.1
  circle A12 centre (10, 411) radius 2.1
  circle A13 centre (160, 411) radius 2.1
  line L0 (640, 401) -> (640, 1000)
  line L1 (640, 1000) -> (0, 1000)
  line L2 (0, 1000) -> (0, 401)
  line L3 (0, 401) -> (640, 401)
sketch "Sketch5 (2)" plane through (643, 0, 0) normal (1, 0, 0) x (0, 1, 0)
  circle A0 centre (630, 603.3333) radius 2.1
  circle A1 centre (10, 410) radius 2.1
  circle A2 centre (630, 990) radius 2.1
  circle A3 centre (320, 990) radius 2.1
  circle A4 centre (480, 990) radius 2.1
  circle A5 centre (500, 410) radius 2.1
  circle A6 centre (10, 603.3333) radius 2.1
  circle A7 centre (630, 410) radius 2.1
  circle A8 centre (160, 990) radius 2.1
  circle A9 centre (10, 796.6667) radius 2.1
  circle A10 centre (10, 990) radius 2.1
  circle A11 centre (200, 410) radius 2.1
  circle A12 centre (630, 796.6667) radius 2.1
  line L0 (640, 400) -> (640, 1000)
  line L1 (640, 1000) -> (0, 1000)
  line L2 (0, 1000) -> (0, 400)
  line L3 (0, 400) -> (640, 400)
sketch "Sketch6 (2)" plane through (-3, 0, 0) normal (-1, 0, 0) x (0, -1, 0)
  circle A0 centre (-370, 410) radius 2.1
  circle A1 centre (-370, 566) radius 2.1
  circle A2 centre (-630, 566) radius 2.1
  circle A3 centre (-10, 990) radius 2.1
  circle A4 centre (-10, 796.6667) radius 2.1
  circle A5 centre (-10, 410) radius 2.1
  circle A6 centre (-630, 410) radius 2.1
  circle A7 centre (-630, 796.6667) radius 2.1
  circle A8 centre (-160, 990) radius 2.1
  circle A9 centre (-480, 990) radius 2.1
  circle A10 centre (-630, 603.3333) radius 2.1
  circle A11 centre (-200, 410) radius 2.1
  circle A12 centre (-10, 603.3333) radius 2.1
  circle A13 centre (-630, 990) radius 2.1
  circle A14 centre (-320, 990) radius 2.1
  line L0 (0, 1000) -> (-640, 1000)
  line L1 (-640, 1000) -> (-640, 400)
  line L2 (-640, 400) -> (0, 400)
  line L3 (0, 400) -> (0, 1000)
component "Frame" placed x (1, 0, 0) y (0, 1, 0) z (0, 0, 1) at (0, 0, 0)
hidden bodies 23
equation "frame_width = 600 mm"
equation "frame_profile = 20 mm"
equation "height = 1000 mm"
equation "pannel_depth = 200 mm"
equation "d44 = frame_width + 2 * frame_profile"
equation "d45 = frame_profile"
equation "d46 = frame_profile"
equation "d47 = frame_profile"
equation "d48 = frame_profile"
equation "d49 = height"
equation "d54 = pannel_depth"
equation "d55 = frame_profile"
equation "d56 = height - frame_width"
equation "d64 = frame_profile / 2"
equation "d65 = frame_profile / 2"
equation "d66 = frame_profile / 2"
equation "d67 = frame_profile"
equation "d68 = ( height - frame_width ) / 2"
equation "d69 = -frame_profile"
equation "d71 = height"
equation "d72 = -frame_profile"
equation "d74 = height"
equation "d75 = -frame_profile"
equation "d77 = height"
equation "d78 = -frame_profile"
equation "d80 = height"
equation "d81 = -frame_profile"
equation "d84 = -frame_profile"
equation "d87 = -frame_profile"
equation "d90 = -frame_profile"
equation "d93 = -frame_profile"
equation "d109 = -frame_profile"
equation "d112 = -frame_profile"
equation "d138 = frame_profile"
equation "hole = 4.2 mm"
equation "d170 = frame_profile / 2"
equation "d171 = frame_profile / 2"
equation "d172 = frame_profile / 2"
equation "d173 = frame_profile / 2"
equation "d174 = hole"
equation "d193 = hole"
equation "d197 = hole"
equation "d200 = frame_profile"
equation "d202 = hole"
equation "d217 = frame_profile"
equation "d218 = frame_profile"
equation "d219 = frame_profile"